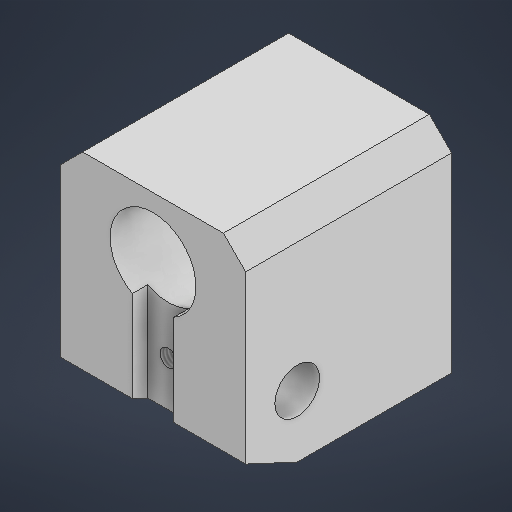
# Autodesk Inventor part: GiaDo
Saved by Autodesk Inventor 2025.4 (Build 294407000, 407)
## iProperties
Created: 2026-05-15
Part Number: GiaDo
Material: Generic
Document SubType Name: Modeling
Designer: VuQuan
Density: 1 g/cm^3
Appearance: Default
Author: VuQuan
Autodesk Inventor part; units mm, degrees
ref_plane "YZ Plane" through (0, 0, 0) normal (1, 0, 0) x (0, 1, 0)
ref_plane "XZ Plane" through (0, 0, 0) normal (0, 1, 0) x (-1, 0, 0)
ref_plane "XY Plane" through (0, 0, 0) normal (0, 0, 1) x (1, 0, 0)
sketch "Sketch1" plane through (0, 0, 0) normal (0, 0, 1) x (1, 0, 0)
  line L0 (-20.5, 62) -> (20.5, 62)
  line L1 (27, 55.5) -> (27, 0)
  line L2 (27, 0) -> (-27, 0)
  line L3 (-27, 0) -> (-27, 55.5)
  line L4 (-27, 55.5) -> (-20.5, 62)
  line L5 (20.5, 62) -> (27, 55.5)
  point P0 (0, 0)
  point P1 (-27, 62)
  point P2 (27, 62)
  point P3 (0, 0)
  dimension "d0" = 62
  dimension "d1" = 6.5
  dimension "d5" = 6.5
  constraints: 12 end point, 4 point on line, 2 equal length, 2 parallel, 1 coincident, 1 horizontal, 1 midpoint, 1 perpendicular
  measures "d0" distance between parallel lines of L0 L2
  measures "d1" distance of L3.end point (-27, 62)
  measures "d5" distance of L0.start point (-27, 62)
extrude "Extrusion1" add sketch "Sketch1" along normal blind 60
chamfer "Chamfer1" distance 7 distance2 15 1 edges at (0, 0, 60) measured on face at (0, 0.5, 60)
sketch "Sketch2" plane through (0, 0, 60) normal (0, 0, 1) x (1, 0, 0)
  line L0 (-27, 0) -> (27, 0) projected
  line L1 (20.5, 62) -> (-20.5, 62) projected
  circle A0 centre (0, 44.5) radius 12.5
  circle A1 centre (0, 44.5) radius 7.5
  line L2 (6, 33.5341) -> (6, 0)
  line L3 (6, 0) -> (-6, 0)
  line L4 (-6, 0) -> (-6, 33.5341)
  line L5 (27, 7) -> (-27, 7) projected
  point P0 (0, 0)
  point P1 (0, 62)
  point P2 (0, 0)
  point P3 (6, 0)
  point P4 (0, 18)
  dimension "d8" = 15
  dimension "d9" = 25
  dimension "d10" = 44.5
  dimension "d11" = 12
  dimension "d21" = 11
  constraints: 6 end point, 3 vertical alignment, 2 centre point, 2 midpoint, 2 perpendicular, 2 point on circle, 1 coincident, 1 collinear, 1 vertical
  measures "d8" diameter of A1
  measures "d9" diameter of A0
  measures "d10" distance from line of L0 A0.centre
  measures "d11" distance between parallel lines of L2 L4
  measures "d21" distance from line of L5 point (0, 18)
extrude "Extrusion2" cut sketch "Sketch2" against normal up to surface (60 mm away) contours A1
extrude "Extrusion3" cut sketch "Sketch2" against normal blind 50 contours A0
extrude "Extrusion4" cut sketch "Sketch2" against normal blind 4.5 contours L4 L5 L2 L0 | L4 A0 L2 L5
sketch "Sketch3" plane through (-27, 0, 0) normal (-1, 0, 0) x (0, 0, 1)
  circle A0 centre (45, 18) radius 6.5
  point P0 (45, 0)
  point P1 (60, 18)
  dimension "d22" = 13
  constraints: 1 centre point, 1 horizontal alignment, 1 vertical alignment
  measures "d22" diameter of A0
extrude "Extrusion5" cut sketch "Sketch3" against normal up to surface (54 mm away)
hole "Hole1" at (0, 18, 60) direction (0, 0, -1) diameter 4.917 end up to surface thread size "M6x1" class "6H" standard "ISO Metric profile"
sketch "Sketch4" plane through (-27, 0, 0) normal (-1, 0, 0) x (0, 0, 1)
  line L0 (0, 0) -> (45, 0) projected
  line L1 (10, 37) -> (10, 52) projected
  line L2 (3.5, 0) -> (3.5, 3.5)
  line L3 (3.5, 3.5) -> (10, 7)
  line L4 (10, 7) -> (16.5, 3.5)
  line L5 (16.5, 3.5) -> (16.5, 0)
  line L6 (10, 7) -> (10, 0)
  point P0 (60, 7)
  point P1 (10, 3.5)
  dimension "d32" = 13
  constraints: 10 end point, 4 point on line, 3 horizontal alignment, 2 perpendicular, 1 equal length, 1 midpoint, 1 vertical
  measures "d32" distance between parallel lines of L5 L2
extrude "Extrusion6" cut sketch "Sketch4" along normal mid plane 13 from surface at -27
equation "\"d5\" = d1"
body "Solid1"
